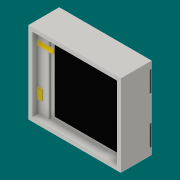
# Autodesk Inventor part: S13360
Saved by Autodesk Inventor 2016 (Build 200138000, 138)
## iProperties
Created: 2016-02-09
Part Number: S13360
Material: ABS Plastic
Document SubType Name: Modeling
Designer: Sawaiz
Density: 1.06 g/cm^3
Appearance: Smooth - White
Author: Sawaiz
Autodesk Inventor part; units mm, degrees
ref_plane "YZ Plane" through (0, 0, 0) normal (1, 0, 0) x (0, 1, 0)
ref_plane "XZ Plane" through (0, 0, 0) normal (0, 1, 0) x (-1, 0, 0)
ref_plane "XY Plane" through (0, 0, 0) normal (0, 0, 1) x (1, 0, 0)
sketch "Sketch1" plane through (0, 0, 0) normal (1, 0, 0) x (0, 1, 0)
  line L0 (-2.175, 1.925) -> (2.175, 1.925)
  line L1 (2.175, 1.925) -> (2.175, -1.925)
  line L2 (2.175, -1.925) -> (-2.175, -1.925)
  line L3 (-2.175, -1.925) -> (-2.175, 1.925)
  line L4 (-2.175, 1.925) -> (2.175, -1.925) construction
  line L5 (2.175, 1.925) -> (-2.175, -1.925) construction
  point P0 (0, 0)
  dimension "d0" = 4.35
  dimension "d1" = 3.85
  constraints: 12 end point, 2 midpoint, 2 parallel, 1 horizontal, 1 perpendicular
  measures "d0" distance of L1.end L2.end
  measures "d1" distance of L0.end L1.end
extrude "Extrusion1" add sketch "Sketch1" along normal blind 1.45
sketch "Sketch2" plane through (1.45, 0, 0) normal (1, 0, 0) x (0, 0, -1)
  line L0 (1.75, -1.5) -> (-1.75, -1.5)
  line L1 (-1.75, -1.5) -> (-1.75, 2)
  line L2 (-1.75, 2) -> (1.75, 2)
  line L3 (1.75, 2) -> (1.75, -1.5)
  line L4 (1.75, -1.5) -> (-1.75, 2) construction
  line L5 (-1.75, -1.5) -> (1.75, 2) construction
  point P0 (0, 0)
  point P1 (0, 0.25)
  dimension "d4" = 0.25
  dimension "d5" = 3.5
  dimension "d6" = 3.5
  constraints: 12 end point, 2 midpoint, 2 parallel, 1 horizontal, 1 perpendicular
  measures "d4" distance of point (0, 0) point (0, 0.25)
  measures "d5" distance of L1.end L2.end
  measures "d6" distance of L0.end L1.end
extrude "Extrusion2" cut sketch "Sketch2" against normal blind 0.4
sketch "Sketch3" plane through (1.05, 0, 0) normal (1, 0, 0) x (0, 0, -1)
  line L0 (1.75, -1.5) -> (-1.75, -1.5) projected
  line L1 (1.75, 2) -> (1.75, -1.5) projected
  line L2 (-1.75, 2) -> (1.75, 2) projected
  line L3 (-1.75, -1.5) -> (-1.75, 2) projected
  line L4 (1.75, 2) -> (-1.75, -1.5) construction
  line L5 (1.5, -1.25) -> (-1.5, -1.25)
  line L6 (-1.5, -1.25) -> (-1.5, 1.75)
  line L7 (-1.5, 1.75) -> (1.5, 1.75)
  line L8 (1.5, 1.75) -> (1.5, -1.25)
  line L9 (1.5, -1.25) -> (-1.5, 1.75) construction
  line L10 (-1.5, -1.25) -> (1.5, 1.75) construction
  point P0 (0, 0)
  point P1 (0, 0.25)
  dimension "d9" = 3
  dimension "d10" = 3
  constraints: 14 end point, 3 midpoint, 2 parallel, 1 horizontal, 1 perpendicular
  measures "d9" distance of L6.end L7.end
  measures "d10" distance of L5.end L6.end
extrude "Extrusion3" add sketch "Sketch3" along normal blind 0.1 contours L5 L6 L7 L8
sketch "Sketch4" plane through (1.45, 0, 0) normal (1, 0, 0) x (0, 0, -1)
  line L0 (1.75, 2) -> (1.75, -1.5) projected
  line L1 (1.75, -1.5) -> (-1.75, -1.5) projected
  line L2 (-1.75, -1.5) -> (-1.75, 2) projected
  line L3 (-1.75, 2) -> (1.75, 2) projected
  line L4 (-1.925, 2.175) -> (-1.925, -2.175) projected
  line L5 (-1.925, -2.175) -> (1.925, -2.175) projected
  line L6 (1.925, -2.175) -> (1.925, 2.175) projected
  line L7 (1.925, 2.175) -> (-1.925, 2.175) projected
  line L8 (-1.75, -1.5) -> (-1.75, 2) projected
  line L9 (-1.75, -1.5) -> (1.75, -1.5)
  line L10 (1.75, -1.5) -> (1.75, -2)
  line L11 (1.75, -2) -> (-1.75, -2)
  line L12 (-1.75, -2) -> (-1.75, -1.5)
  point P0 (0, 0)
  dimension "d13" = 0.5
  constraints: 8 end point, 2 parallel, 1 horizontal, 1 perpendicular
  measures "d13" distance of L9.end L10.end
extrude "Extrusion4" cut sketch "Sketch4" against normal blind 0.3 contours L10 L11 L12 L1
sketch "Sketch5" plane through (1.15, 0, 0) normal (1, 0, 0) x (0, 0, -1)
  line L0 (1.75, -2) -> (-1.75, -2) projected
  line L1 (-1.2563, -2) -> (-1.0563, -2)
  line L2 (-1.0563, -2) -> (-1.0563, -1.25)
  line L3 (-1.0563, -1.25) -> (-1.2563, -1.25)
  line L4 (-1.2563, -1.25) -> (-1.2563, -2)
  line L5 (0.6375, -2) -> (1.1375, -2)
  line L6 (1.1375, -2) -> (1.1375, -1.8)
  line L7 (1.1375, -1.8) -> (0.6375, -1.8)
  line L8 (0.6375, -1.8) -> (0.6375, -2)
  line L9 (-1.5, -1.25) -> (1.5, -1.25) projected
  point P0 (0, 0)
  dimension "d16" = 0.2
  dimension "d17" = 0.5
  dimension "d18" = 0.2
  constraints: 16 end point, 4 parallel, 2 horizontal, 2 perpendicular, 2 point on line, 1 collinear
  measures "d16" distance of L5.end L6.end
  measures "d17" distance of L6.end L7.end
  measures "d18" distance between parallel lines of L4 L2
extrude "Extrusion5" add sketch "Sketch5" along normal blind 0.05
sketch "Sketch6" plane through (0, 0, 0) normal (-1, 0, 0) x (0, 0, 1)
  line L0 (1.925, -2.175) -> (1.925, 2.175) projected
  line L1 (1.925, 2.175) -> (-1.925, 2.175) projected
  line L2 (-1.925, 2.175) -> (-1.925, -2.175) projected
  line L3 (-1.925, -2.175) -> (1.925, -2.175) projected
  line L4 (1.6, 2.175) -> (0.6, 2.175)
  line L5 (0.6, 2.175) -> (0.6, -2.075)
  line L6 (0.6, -2.075) -> (1.6, -2.075)
  line L7 (1.6, -2.075) -> (1.6, 2.175)
  line L8 (-1.6, -2.075) -> (-0.6, -2.075)
  line L9 (-0.6, -2.075) -> (-0.6, 2.175)
  line L10 (-0.6, 2.175) -> (-1.6, 2.175)
  line L11 (-1.6, 2.175) -> (-1.6, -2.075)
  line L12 (1.925, 2.175) -> (-1.925, 2.175) projected
  point P0 (0, 0)
  point P1 (1.1, -2.075)
  point P2 (-1.1, -2.075)
  dimension "d21" = 1
  dimension "d22" = 1
  dimension "d23" = 4.25
  dimension "d24" = 4.25
  dimension "d25" = 1.1
  dimension "d26" = 1.1
  constraints: 16 end point, 4 parallel, 2 collinear, 2 horizontal, 2 midpoint, 2 perpendicular
  measures "d21" distance of L8.start L8.end
  measures "d22" distance of L5.end L6.end
  measures "d23" distance of L6.end L4.start
  measures "d24" distance between parallel lines of L8 L10
  measures "d25" horizontal distance of point (0, 0) point (-1.1, -2.075)
  measures "d26" horizontal distance of point (1.1, -2.075) point (0, 0)
extrude "Extrusion6" cut sketch "Sketch6" against normal blind 0.1 contours L7 L6 L5 L1 | L1 L9 L8 L11
sketch "Sketch7" plane through (0.1, 0, 0) normal (-1, 0, 0) x (0, 0, 1)
  line L0 (0.6, 2.175) -> (1.6, 2.175) projected
  line L1 (0.6, -2.075) -> (0.6, 2.175) projected
  line L2 (1.6, -2.075) -> (0.6, -2.075) projected
  line L3 (1.6, 2.175) -> (1.6, -2.075) projected
  line L4 (-0.6, -2.075) -> (-1.6, -2.075) projected
  line L5 (-0.6, 2.175) -> (-0.6, -2.075) projected
  line L6 (-1.6, 2.175) -> (-0.6, 2.175) projected
  line L7 (-1.6, -2.075) -> (-1.6, 2.175) projected
  point P0 (0, 0)
extrude "Extrusion7" add sketch "Sketch7" along normal up to surface (0.1 mm away) separate body
sketch "Sketch8" plane through (0, 0, 0) normal (-1, 0, 0) x (0, 0, 1)
  circle A0 centre (-0.3, 0) radius 0.1
  point P0 (0, 0)
  dimension "d31" = 0.2
  dimension "d32" = 0.3
  constraints: 1 centre point
  measures "d31" diameter of A0
  measures "d32" distance of point (0, 0) A0.centre
extrude "Extrusion8" cut sketch "Sketch8" against normal blind 0.1 bodies 1
equation "\"d26\" = d25"
body "Solid1"
body "Solid2"
